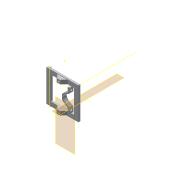
# Autodesk Inventor part: 40_XY_Stage_Clamp_Slide
Saved by Autodesk Inventor 2019 (Build 230136000, 136)
## iProperties
Created: 2019-04-29
Part Number: 40_XY_Stage_Clamp_Slide
Material: Generic
Document SubType Name: Modeling
Designer: diederichbenedict
Density: 1 g/cm^3
Appearance: White
Author: diederichbenedict
Autodesk Inventor part; units mm, degrees
ref_plane "YZ Plane" through (0, 0, 0) normal (1, 0, 0) x (0, 1, 0)
ref_plane "XZ Plane" through (0, 0, 0) normal (0, 1, 0) x (-1, 0, 0)
ref_plane "XY Plane" through (0, 0, 0) normal (0, 0, 1) x (1, 0, 0)
ref_plane "Work Plane1" through (0, -100, 0) normal (0, 0, 1) x (1, 0, 0)
sketch "Sketch1" plane through (0, -100, 0) normal (0, 0, 1) x (1, 0, 0)
  circle A0 centre (-10.9624, 74.9427) radius 1.35 construction
  circle A1 centre (11.0376, 74.9427) radius 1.35 construction
  circle A2 centre (-0.6624, 100.2177) radius 3 construction
  arc A3 (9.6715, 71.4427) -> (-9.5963, 71.4427) centre (0.0376, 55.9427) ccw construction
  arc A4 (9.6715, 71.4427) -> (-9.5963, 71.4427) centre (0.0376, 55.9427) ccw construction
  arc A5 (9.6715, 71.4427) -> (-9.5963, 71.4427) centre (0.0376, 55.9427) ccw projected
  arc A6 (9.6715, 71.4427) -> (-9.5963, 71.4427) centre (0.0376, 55.9427) ccw projected
  arc A7 (9.6715, 71.4427) -> (-9.5963, 71.4427) centre (0.0376, 55.9427) ccw projected
  circle A8 centre (0.0376, 55.9427) radius 18.25
  line L0 (9.6715, 71.4427) -> (14.0876, 71.4427) projected
  line L1 (14.0876, 71.4427) -> (14.0876, 109.7677) projected
  line L2 (14.0876, 109.7677) -> (-12.6124, 109.7677) projected
  line L3 (-12.6124, 109.7677) -> (-12.6124, 71.4427) projected
  line L4 (-12.6124, 71.4427) -> (-9.5963, 71.4427) projected
  circle A9 centre (-10.9624, 74.9427) radius 1.35 projected
  circle A10 centre (11.0376, 74.9427) radius 1.35 projected
  circle A11 centre (-0.6624, 100.2177) radius 3 projected
  line L5 (9.6715, 71.4427) -> (14.0876, 71.4427) projected
  line L6 (14.0876, 71.4427) -> (14.0876, 109.7677) projected
  line L7 (14.0876, 109.7677) -> (-12.6124, 109.7677) projected
  line L8 (-12.6124, 109.7677) -> (-12.6124, 71.4427) projected
  line L9 (-12.6124, 71.4427) -> (-9.5963, 71.4427) projected
  circle A12 centre (19.8876, 36.0427) radius 1.75 construction
  circle A13 centre (-19.9624, 36.0427) radius 1.75 construction
  circle A14 centre (-19.9624, 76.0427) radius 1.75 construction
  circle A15 centre (19.8876, 76.0427) radius 1.6 construction
  line L10 (25.0376, 30.9427) -> (25.0376, 80.9427) construction
  arc A16 (14.7376, 33.8211) -> (17.7376, 30.8211) centre (17.7376, 33.8211) ccw construction
  line L11 (-24.9624, 30.9427) -> (25.0376, 30.9427) construction
  line L12 (-24.9624, 80.9427) -> (-24.9624, 30.9427) construction
  line L13 (25.0376, 80.9427) -> (-24.9624, 80.9427) construction
  line L14 (25.0376, 48.675) -> (25.0376, 30.9427) construction
  line L15 (25.0376, 30.9427) -> (-24.9624, 30.9427)
  line L16 (-24.9624, 30.9427) -> (-24.9624, 80.9427)
  line L17 (-24.9624, 80.9427) -> (25.0376, 80.9427)
  line L18 (25.0376, 80.9427) -> (25.0376, 30.9427)
  line L19 (25.0376, 30.9427) -> (-24.9624, 80.9427) construction
  line L20 (-24.9624, 30.9427) -> (25.0376, 80.9427) construction
  point P0 (0, 100)
  point P1 (-12.6124, 40.4427)
  point P2 (15.0876, 40.4427)
  constraints: 22 end point, 5 centre point, 3 horizontal, 2 midpoint, 2 parallel, 2 point on circle, 2 vertical, 1 coincident, 1 collinear, 1 perpendicular, 1 point on line, 19 other
extrude "Extrusion1" add sketch "Sketch1" along normal blind 3 contours L0 L1 L17 L18 L15 L16 L3 L4 A8 | A5 L4 L3 L17 L1 L0 | A9 | A10
sketch "Sketch2" plane through (0.0376, -44.0573, 0) normal (0, 0, -1) x (-1, 0, 0)
  circle A0 centre (11, -19) radius 1.35 projected
  point P0 (0.0376, 44.0573)
ref_plane "Work Plane2" through (-19.9624, -69.0573, 0) normal (-1, 0, 0) x (0, 0, 1)
sketch "Sketch3" plane through (-19.9624, -69.0573, 0) normal (-1, 0, 0) x (0, 0, 1)
  line L0 (0.8019, 0) -> (0.8019, 4.9825)
  arc A0 (0.8019, 7.15) -> (0.8019, 3.05) centre (0.8019, 5.1) ccw
  line L1 (0.8019, 3.05) -> (0.8019, 7.15)
  circle A1 centre (-29.6088, 5.1) radius 1.5
  point P0 (0, 69.0573)
  dimension "d8" = 4.1
  dimension "d9" = 2.05
  constraints: 4 end point, 2 centre point, 2 point on circle, 2 point on line, 1 collinear, 1 vertical, 2 other
  measures "d8" distance of L1.end L1.start
  measures "d9" radius of A0
revolve "Revolution1" cut sketch "Sketch3" angle 360 about axis through (-19.9624, -69.0573, 0.8019) along (0, 1, 0) contours A0 L1 L0
pattern_linear "Rectangular Pattern1" count 2 spacing 40 along (0, 1, 0) count 2 spacing 40 along (1, 0, 0) of "Revolution1"
sketch "Sketch4" plane through (0.0376, -44.0573, 3) normal (0, 0, 1) x (1, 0, 0)
  circle A0 centre (0, 0) radius 18.25 projected
  circle A1 centre (0, 0) radius 21.25
  line L0 (3, 24.25) -> (-3, 24.25)
  line L1 (-3, 24.25) -> (-3, 18.25)
  line L2 (-3, 18.25) -> (3, 18.25)
  line L3 (3, 18.25) -> (3, 24.25)
  line L4 (3, 24.25) -> (-3, 18.25) construction
  line L5 (-3, 24.25) -> (3, 18.25) construction
  line L6 (3, -18.25) -> (-3, -18.25)
  line L7 (-3, -18.25) -> (-3, -24.25)
  line L8 (-3, -24.25) -> (3, -24.25)
  line L9 (3, -24.25) -> (3, -18.25)
  line L10 (3, -18.25) -> (-3, -24.25) construction
  line L11 (-3, -18.25) -> (3, -24.25) construction
  point P0 (-0.0376, 44.0573)
  point P1 (0, 21.25)
  point P2 (0, -21.25)
  dimension "d17" = 3
  dimension "d18" = 6
  dimension "d19" = 6
  dimension "d20" = 6
  dimension "d21" = 6
  constraints: 24 end point, 4 midpoint, 4 parallel, 2 horizontal, 2 perpendicular, 2 point on circle, 1 centre point
  measures "d17" radial gap between concentric circles of A0 A1
  measures "d18" distance of L2.end L1.end
  measures "d19" distance of L1.end L0.end
  measures "d20" distance of L8.end L7.end
  measures "d21" distance of L7.end L6.end
extrude "Extrusion2" add sketch "Sketch4" along normal blind 6 contours L2 L1 A1 L3 | L6 L9 A1 L7 | L1 L0 L3 A1 | L9 L8 L7 A1
ref_plane "Work Plane3" through (14.7376, -44.0573, -61.6) normal (0, 1, 0) x (-1, 0, 0)
ref_plane "Work Plane4" through (0.0376, -44.0573, -9.7) normal (0, 0, 1) x (-0.9939, 0.11, 0)
chamfer "Chamfer1" distance 5 angle 45 4 edges at (-2.9624, -22.8073, 3) (3.0376, -65.3073, 3) (3.0376, -22.8073, 3) (-2.9624, -65.3073, 3)
sketch "Sketch8" plane through (0.0376, -44.0573, 0) normal (0, 0, -1) x (-1, 0, 0)
  circle A0 centre (0, 0) radius 18.25 projected
  circle A1 centre (0, 0) radius 21
  line L0 (-18.25, -18.25) -> (18.25, -18.25)
  line L1 (18.25, -18.25) -> (18.25, 18.25)
  line L2 (18.25, 18.25) -> (-18.25, 18.25)
  line L3 (-18.25, 18.25) -> (-18.25, -18.25)
  line L4 (-18.25, -18.25) -> (18.25, 18.25) construction
  line L5 (18.25, -18.25) -> (-18.25, 18.25) construction
  point P0 (0.0376, 44.0573)
  dimension "d46" = 42
  constraints: 12 end point, 2 midpoint, 2 parallel, 1 centre point, 1 coincident, 1 horizontal, 1 perpendicular
  measures "d46" diameter of A1
extrude "Extrusion4" cut sketch "Sketch8" against normal up to surface (3 mm away) contours A0 | L1 A1 L0 A0 | A0 L2 A1 L1 | A0 L3 A1 L2 | L0 A1 L3 A0 | L1 L0 A1 | A1 L2 L1 | A1 L3 L2 | L0 L3 A1
sketch "Sketch13" plane through (0.0376, -44.0573, 9) normal (0, 0, 1) x (1, 0, 0)
  line L0 (3, 24.25) -> (-3, 24.25) projected
  line L1 (-3, 24.25) -> (-3, 18.25) projected
  line L2 (-3, 18.25) -> (3, 18.25) projected
  line L3 (3, 18.25) -> (3, 24.25) projected
  line L4 (3, -18.25) -> (-3, -18.25) projected
  line L5 (-3, -18.25) -> (-3, -24.25) projected
  line L6 (-3, -24.25) -> (3, -24.25) projected
  line L7 (3, -24.25) -> (3, -18.25) projected
  circle A0 centre (0, 21.25) radius 3
  circle A1 centre (0, -21.25) radius 3
  point P0 (-0.0376, 44.0573)
  constraints: 6 tangent, 2 centre point
hole "Hole1" at (0.0376, -22.8073, 9) at (0.0376, -65.3073, 9) direction (0, 0, -1) diameter 2.8 depth 14 tip angle 118
sketch "Sketch14" plane through (0, -100, 0) normal (0, 0, -1) x (-1, 0, 0)
  circle A0 centre (-0.0376, 34.6927) radius 1.4 projected
  line L0 (-3.0376, 37.6927) -> (2.9624, 37.6927) projected
  line L1 (2.9624, 37.6927) -> (2.9624, 31.6927) projected
  line L2 (2.9624, 31.6927) -> (-3.0376, 31.6927) projected
  line L3 (-3.0376, 31.6927) -> (-3.0376, 37.6927) projected
  line L4 (-3.0376, 31.6927) -> (2.9624, 31.6927)
  line L5 (2.9624, 31.6927) -> (2.9624, 37.6927)
  line L6 (2.9624, 37.0253) -> (-3.0376, 37.0253)
  line L7 (-3.0376, 37.0253) -> (-3.0376, 31.0253)
  circle A1 centre (-0.0376, 34.6927) radius 1.4
  line L8 (-11.1896, 38.2279) -> (-4.8641, 38.2279) construction
  line L9 (-4.8641, 38.2279) -> (-4.8641, 44.2875) construction
  line L10 (-4.8641, 44.2875) -> (-11.1896, 44.2875) construction
  line L11 (-11.1896, 44.2875) -> (-11.1896, 38.2279) construction
  circle A2 centre (-7.8641, 41.2875) radius 1.4 construction
  line L12 (-11.1896, 38.2279) -> (-14.1896, 38.2279)
  line L13 (-14.1896, 38.2279) -> (-14.1896, 45.2279)
  line L14 (-14.1896, 45.2279) -> (-11.1896, 45.2279)
  line L15 (-11.1896, 45.2279) -> (-11.1896, 38.2279)
  line L16 (-11.1896, 45.2279) -> (-11.1896, 46.6199) construction
  line L17 (-11.1896, 46.6199) -> (-2.5633, 49.9064) construction
  line L18 (-2.5633, 49.9064) -> (-2.5633, 52.6062) construction
  spline S0 degree 3 poles (-11.1896, 45.2279) (-11.1896, 46.6199) (-2.5633, 49.9064) (-2.5633, 52.6062) knots 1 1 1 1 2 2 2 2
  line L19 (-14.1896, 45.2279) -> (-14.1896, 48.0119) construction
  line L20 (-14.1896, 48.0119) -> (-3.6365, 49.4975) construction
  line L21 (-3.6365, 49.4975) -> (-3.6365, 56.3825) construction
  spline S1 degree 3 poles (-14.1896, 45.2279) (-14.1896, 48.0119) (-3.6365, 49.4975) (-3.6365, 56.3825) knots 1 1 1 1 2 2 2 2
  line L22 (-3.6365, 56.3825) -> (-2.5633, 56.3825)
  line L23 (-2.5633, 56.3825) -> (-2.5633, 52.6062)
  point P0 (0, 100)
  dimension "d62" = 3
  dimension "d63" = 7
  constraints: 28 end point, 6 parallel, 4 horizontal, 4 perpendicular, 4 vertical, 2 centre point, 1 coincident, 1 concentric, 1 point on line, 6 other
  measures "d62" distance of L13.end L14.end
  measures "d63" distance of L12.end L13.end
extrude "Extrusion7" add sketch "Sketch14" against normal blind 6 contours L12 L13 L14 L15 | L14 S1 L22 L23 S0
sketch "Sketch15" plane through (11.1896, -61.7721, 0) normal (-1, 0, 0) x (0, 0, 1)
  line L0 (0, 0) -> (0, 7) projected
  line L1 (0, 0) -> (6, 0) projected
  line L2 (6, 7) -> (6, 0) projected
  line L3 (0, 7) -> (6, 7) projected
  circle A0 centre (3, 4) radius 3
  point P0 (0, 61.7721)
  constraints: 3 tangent, 1 centre point
hole "Hole2" at (11.1896, -57.7721, 3) direction (1, 0, 0) diameter 3 depth 4 tip angle 118
mirror "Mirror2" about plane through (14.7376, -44.0573, -61.6) normal (0, 1, 0) of "Extrusion7", "Hole2"
body "Solid1"
